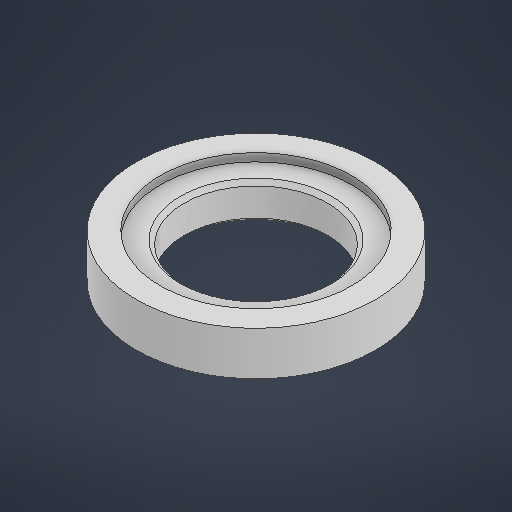
# Autodesk Inventor part: clutch
Saved by Autodesk Inventor 2025.2 (Build 292293000, 293)
## iProperties
Created: 2025-04-19
Part Number: clutch
Material: Generic
Document SubType Name: Modeling
Designer: klawy
Density: 1 g/cm^3
Appearance: Default
Author: klawy
Autodesk Inventor part; units mm, degrees
ref_plane "YZ Plane" through (0, 0, 0) normal (1, 0, 0) x (0, 1, 0)
ref_plane "XZ Plane" through (0, 0, 0) normal (0, 1, 0) x (-1, 0, 0)
ref_plane "XY Plane" through (0, 0, 0) normal (0, 0, 1) x (1, 0, 0)
sketch "Sketch2" plane through (0, 0, 0) normal (0, 0, 1) x (1, 0, 0)
  line L0 (9, 0) -> (15, 0)
  line L1 (15, 0) -> (15, 2.5)
  line L2 (15, 2.5) -> (9, 2.5)
  line L3 (9, 2.5) -> (9, 0)
  line L4 (15, 2.5) -> (12, 2.5)
  line L5 (12, 2.5) -> (12, 5.5)
  line L6 (12, 5.5) -> (15, 5.5)
  line L7 (15, 5.5) -> (15, 2.5)
  line L8 (0, -9.1355) -> (0, 9.1355) construction
  line L9 (15, 2.5) -> (19, 2.5)
  line L10 (19, 2.5) -> (19, 0)
  line L11 (19, 0) -> (15, 0)
  line L12 (15, 0) -> (15, 2.5)
  line L13 (9, 2.5) -> (12, 2.5)
  line L14 (12, 2.5) -> (12, 4.5)
  line L15 (12, 4.5) -> (9, 4.5)
  line L16 (9, 4.5) -> (9, 2.5)
  point P0 (0, 0)
  dimension "d4" = 9
  dimension "d5" = 6
  dimension "d6" = 2.5
  dimension "d7" = 3
  dimension "d8" = 3
  dimension "d14" = 19
  dimension "d15" = 1
  constraints: 34 end point, 8 parallel, 4 horizontal, 4 perpendicular, 3 point on line, 1 midpoint, 1 vertical
  measures "d4" distance from line of point (0, 0) L3
  measures "d5" distance between parallel lines of L1 L3
  measures "d6" distance from line of L0.end L2
  measures "d7" distance of L5.end L6.end
  measures "d8" distance between parallel lines of L6 L2
  measures "d14" distance from line of point (0, 0) L10
  measures "d15" distance between parallel lines of L6 L15
revolve "Revolution1" add sketch "Sketch2" angle 360 about axis through (0, -9.1355, 0) along (0, 1, 0) contours L3 L2 L1 L0 | L16 L15 L5 L2 | L2 L5 L6 L7
chamfer "Chamfer1" distance 0.5 angle 45 2 edges at (-9, 0, 0) (-9, 4.5, 0)
body "Solid1"
